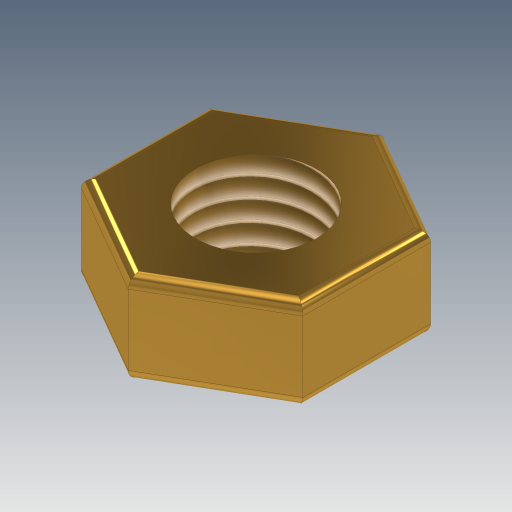
# Autodesk Inventor part: Nut_M3_Brass
Saved by Autodesk Inventor 2024 (Build 280153000, 153)
## iProperties
Created: 2023-06-05
Part Number: Nut_M3_Brass
Material: Brass
Document SubType Name: Modeling
Designer: schanen
Density: 8.49 g/cm^3
Appearance: Brass - Polished
Author: schanen
Autodesk Inventor part; units mm, degrees
ref_plane "YZ Plane" through (0, 0, 0) normal (1, 0, 0) x (0, 1, 0)
ref_plane "XZ Plane" through (0, 0, 0) normal (0, 1, 0) x (-1, 0, 0)
ref_plane "XY Plane" through (0, 0, 0) normal (0, 0, 1) x (1, 0, 0)
sketch "Sketch1" plane through (0, 0, 0) normal (0, 1, 0) x (-1, 0, 0)
  line L0 (2.75, 1.5877) -> (2.75, -1.5877)
  line L1 (2.75, -1.5877) -> (0, -3.1754)
  line L2 (0, -3.1754) -> (-2.75, -1.5877)
  line L3 (-2.75, -1.5877) -> (-2.75, 1.5877)
  line L4 (-2.75, 1.5877) -> (0, 3.1754)
  line L5 (0, 3.1754) -> (2.75, 1.5877)
  circle A0 centre (0, 0) radius 1.5
  dimension "d0" = 5.5
  dimension "d1" = 3
  constraints: 12 end point, 2 coincident, 1 centre point, 1 vertical alignment, 13 other
  measures "d0" distance between parallel lines of L3 L0
  measures "d1" diameter of A0
extrude "Extrusion1" add sketch "Sketch1" along normal blind 2.25
fillet "Fillet1" radius 0.25 12 edges at (2.75, 2.25, 0) (1.375, 2.25, 2.3816) (-1.375, 2.25, 2.3816) (-2.75, 2.25, 0) (-1.375, 2.25, -2.3816) (1.375, 2.25, -2.3816) (2.75, 0, 0) (1.375, 0, 2.3816) (-1.375, 0, 2.3816) (-2.75, 0, 0) (-1.375, 0, -2.3816) (1.375, 0, -2.3816)
thread "Thread1" size "M3x0.5" class "6H" standard "ISO Metric profile" length 11.5
body "Solid1"
